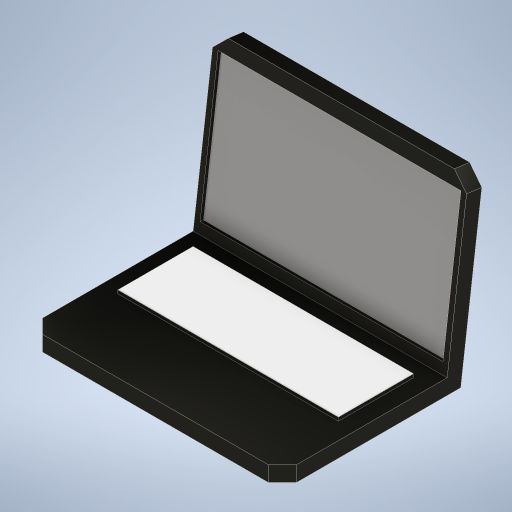
# Autodesk Inventor part: Laptop
Saved by Autodesk Inventor 2024 (Build 280153000, 153)
## iProperties
Created: 2024-01-18
Part Number: Laptop
Material: PBT Plastic
Document SubType Name: Modeling
Designer: ASUS
Density: 1.31 g/cm^3
Appearance: Gunmetal
Author: ASUS
Autodesk Inventor part; units mm, degrees
ref_plane "YZ Plane" through (0, 0, 0) normal (1, 0, 0) x (0, 1, 0)
ref_plane "XZ Plane" through (0, 0, 0) normal (0, 1, 0) x (-1, 0, 0)
ref_plane "XY Plane" through (0, 0, 0) normal (0, 0, 1) x (1, 0, 0)
sketch "Sketch1" plane through (0, 0, 0) normal (1, 0, 0) x (0, 1, 0)
  line L0 (0, 0) -> (22, 0)
  line L1 (22, 0) -> (22, -255)
  line L2 (22, -255) -> (0, -255)
  line L3 (0, -255) -> (0, 0)
  line L4 (0, -255) -> (2.8219, -233.1817)
  line L5 (2.8219, -233.1817) -> (255.7155, -265.8902)
  line L6 (255.7155, -265.8902) -> (252.8936, -287.7085)
  line L7 (252.8936, -287.7085) -> (0, -255)
  point P0 (22, -235.6622)
  dimension "d0" = 22
  dimension "d1" = 255
  dimension "d2" = 22
  dimension "d3" = 255
  constraints: 16 end point, 4 parallel, 2 perpendicular, 1 horizontal
  measures "d0" distance between parallel lines of L3 L1
  measures "d1" distance between parallel lines of L2 L0
  measures "d2" distance of L2.end L4.end
  measures "d3" distance of L4.end L5.end
extrude "Extrusion1" add sketch "Sketch1" along normal blind 363.4
chamfer "Chamfer1" distance 20 angle 45 4 edges at (363.4, 254.3045, -276.7993) (0, 254.3045, -276.7993) (363.4, 11, 0) (0, 11, 0)
sketch "Sketch2" plane through (0, 22, -235.6622) normal (0, 0.1282685, 0.9917395) x (1, 0, 0)
  line L0 (8, 215.6622) -> (355.4, 215.6622)
  line L1 (355.4, 215.6622) -> (355.4, 15)
  line L2 (355.4, 15) -> (8, 15)
  line L3 (8, 15) -> (8, 215.6622)
  line L4 (0, 215.6622) -> (0, 0) projected
  line L5 (363.4, 215.6622) -> (363.4, 0) projected
  line L6 (20, 235.6622) -> (343.4, 235.6622) projected
  line L7 (0, 0) -> (363.4, 0) projected
  point P0 (0, -52.0463)
  dimension "d9" = 8
  dimension "d10" = 8
  dimension "d11" = 20
  dimension "d12" = 15
  constraints: 8 end point, 2 parallel, 1 horizontal, 1 perpendicular
  measures "d9" distance between parallel lines of L4 L3
  measures "d10" distance between parallel lines of L5 L1
  measures "d11" distance between parallel lines of L6 L0
  measures "d12" distance between parallel lines of L7 L2
extrude "Extrusion2" cut sketch "Sketch2" against normal blind 5
sketch "Sketch4" plane through (0, 22, -235.6622) normal (0, 1, 0) x (1, 0, 0)
  line L0 (24, -24.076) -> (339.4, -24.076)
  line L1 (339.4, -24.076) -> (339.4, -131.6622)
  line L2 (339.4, -131.6622) -> (24, -131.6622)
  line L3 (24, -131.6622) -> (24, -24.076)
  line L4 (355.4, 1.924) -> (8, 1.924) projected
  line L5 (0, 0) -> (0, -215.6622) projected
  line L6 (363.4, 0) -> (363.4, -215.6622) projected
  line L7 (20, -235.6622) -> (343.4, -235.6622) projected
  dimension "d15" = 26
  dimension "d16" = 24
  dimension "d17" = 24
  dimension "d18" = 104
  constraints: 8 end point, 2 parallel, 1 horizontal, 1 perpendicular
  measures "d15" distance between parallel lines of L4 L0
  measures "d16" distance between parallel lines of L5 L3
  measures "d17" distance between parallel lines of L6 L1
  measures "d18" distance between parallel lines of L7 L2
extrude "Extrusion3" add sketch "Sketch4" along normal blind 5
body "Solid1"
